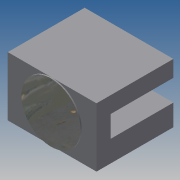
# Autodesk Inventor part: endcapTarget
Saved by Autodesk Inventor 2014 SP1 (Build 180222100, 222)
## iProperties
Created: 2014-08-28
Part Number: endcapTarget
Material: Generic
Document SubType Name: Modeling
Designer: Dave
Density: 1 g/cm^3
Appearance: Default
Author: Dave
Autodesk Inventor part; units mm, degrees
ref_plane "YZ Plane" through (0, 0, 0) normal (1, 0, 0) x (0, 1, 0)
ref_plane "XZ Plane" through (0, 0, 0) normal (0, 1, 0) x (-1, 0, 0)
ref_plane "XY Plane" through (0, 0, 0) normal (0, 0, 1) x (1, 0, 0)
sketch "Sketch1" plane through (0, 0, 0) normal (1, 0, 0) x (0, 1, 0)
  line L0 (18.0976, -11.9743) -> (30.7976, -11.9743)
  line L1 (30.7976, -11.9743) -> (30.7976, -28.4843)
  line L2 (18.0976, -28.4843) -> (18.0976, -11.9743)
  line L3 (27.2855, -28.4843) -> (27.2855, -15.0223)
  line L4 (27.2855, -15.0223) -> (22.6756, -15.0223)
  line L5 (22.6756, -15.0223) -> (22.6756, -28.4843)
  line L6 (30.7976, -28.4843) -> (27.2855, -28.4843)
  line L7 (22.6756, -28.4843) -> (18.0976, -28.4843)
  point P0 (0, 0)
  dimension "d0" = 12.7
  dimension "d1" = 16.51
  dimension "d14" = 3.048
  constraints: 16 end point, 4 parallel, 4 perpendicular, 1 horizontal
  measures "d0" distance of L1.end L2.start
  measures "d1" distance of L0.end L1.end
  measures "d14" distance between parallel lines of L4 L0
extrude "Extrusion1" add sketch "Sketch1" along normal blind 19.05
sketch "Sketch2" plane through (0, 18.0976, -28.4843) normal (0, -1, 0) x (1, 0, 0)
  circle A0 centre (9.525, 5.8867) radius 2.6491
  point P0 (0, 28.4843)
  constraints: 1 centre point
hole "Hole1" at (9.525, 18.0976, -22.5976) direction (0, 1, 0) diameter 3.302 depth 7.62 tip angle 118 thread size "8-32 UNC" class "2B" standard "ANSI Unified Screw Threads"
sketch "Sketch3" plane through (0, 18.0976, -11.9743) normal (0, 0, 1) x (1, 0, 0)
  circle A0 centre (9.525, 6.35) radius 6.35
  point P0 (0, -18.0976)
  dimension "d11" = 12.7
  constraints: 1 centre point
  measures "d11" diameter of A0
extrude "Extrusion2" add sketch "Sketch3" along normal blind 0.254
body "Solid1"
